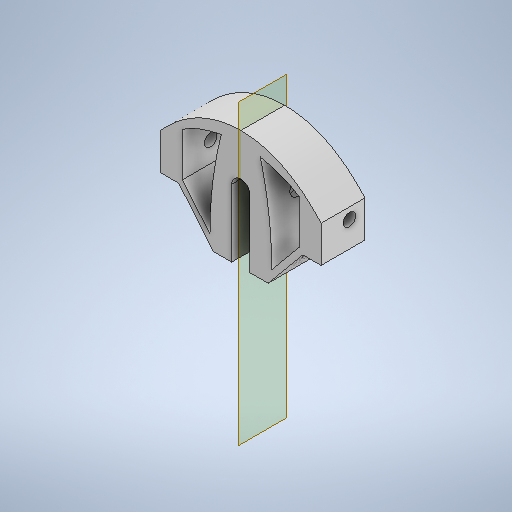
# Autodesk Inventor part: 5th Wheel Body
Saved by Autodesk Inventor 2025 (Build 290162000, 162)
## iProperties
Created: 2024-06-19
Part Number: 5th Wheel Body
Material: 일반
Document SubType Name: Modeling
Designer: unney
Density: 1 g/cm^3
Appearance: 기본값
Author: unney
Autodesk Inventor part; units mm, degrees
ref_plane "YZ Plane" through (0, 0, 0) normal (1, 0, 0) x (0, 1, 0)
ref_plane "XZ Plane" through (0, 0, 0) normal (0, 1, 0) x (-1, 0, 0)
ref_plane "XY Plane" through (0, 0, 0) normal (0, 0, 1) x (1, 0, 0)
sketch "스케치1" plane through (0, 0, 0) normal (0, 0, 1) x (1, 0, 0)
  arc A0 (0, 12.5) -> (-12.5, 0) centre (0, 0) ccw
  line L0 (0, 220.6094) -> (0, -371.145)
  line L1 (-77.086, -220) -> (-110, -35)
  line L2 (-110, -35) -> (-110, 15)
  spline S0 degree 2 poles (-110, 15) (-61.239, 69.4656) (0, 70) knots 0 0 0 1 1 1
  line L3 (-29.7943, 69.74) -> (29.7943, 70.26) construction
  line L4 (-12.5, 0) -> (-12.5, -190)
  line L5 (-12.5, -190) -> (-29.9689, -220)
  line L6 (-29.9689, -220) -> (-77.086, -220)
  arc A1 (12.5, 0) -> (0, 12.5) centre (0, 0) ccw
  line L7 (77.086, -220) -> (110, -35)
  line L8 (110, -35) -> (110, 15)
  spline S1 degree 2 poles (110, 15) (61.239, 69.4656) (0, 70) knots 0 0 0 1 1 1
  line L9 (29.7943, 69.74) -> (-29.7943, 70.26) construction
  line L10 (12.5, 0) -> (12.5, -190)
  line L11 (12.5, -190) -> (29.9689, -220)
  line L12 (29.9689, -220) -> (77.086, -220)
  point P0 (1.2114, -68.8044)
  point P1 (23.5091, 68.2027)
  point P2 (-23.4485, 67.5354)
  point P3 (-1.2114, -68.8044)
  point P4 (-23.5091, 68.2027)
  point P5 (23.4485, 67.5354)
  point P6 (0, 70)
  dimension "d0" = 25
  dimension "d3" = 110
  dimension "d4" = 50
  dimension "d5" = 190
  dimension "d8" = 70
  dimension "d25" = 290
  constraints: 26 end point, 11 symmetric about line, 4 midpoint, 4 point on circle, 2 centre point, 2 point on line, 2 vertical, 1 coincident, 1 horizontal, 1 parallel, 1 perpendicular, 15 other
  measures "d0" diameter of A0
  measures "d3" distance between parallel lines of L0 L2
  measures "d4" distance of L2.end L1.end
  measures "d5" distance of L4.end L4.start
  measures "d8" distance of point (0, 0) point (0, 70)
  measures "d25" distance from line of L12 point (0, 70)
extrude "Wheel Body Initial Extrusion" add sketch "스케치1" along normal mid plane 60
sketch "스케치4" plane through (-12.5, -190, 30) normal (1, 0, 0) x (0, 0, -1)
  line L0 (60, 190) -> (0, 190) projected
  line L1 (60, 190) -> (60, 0) projected
  line L2 (60, 0) -> (0, 0) projected
  line L3 (0, 0) -> (0, 190) projected
  line L4 (0, 190) -> (0, -93.6851)
  line L5 (23, 50) -> (10, 50)
  line L6 (10, 50) -> (10, -48.4584)
  line L7 (10, -10.6044) -> (23, -10.6044)
  line L8 (23, -10.6044) -> (23, -50.5115)
  line L9 (23, -50.5115) -> (0, -50.5115)
  line L10 (53, -93.6851) -> (53, 276.7845)
  line L11 (53, 190) -> (0, 190)
  line L12 (53, 259.8429) -> (0, 259.8429)
  line L13 (0, 259.8429) -> (0, 0)
  point P0 (30, 190)
  dimension "d18" = 13
  dimension "d19" = 140
  dimension "d20" = 7
  constraints: 20 end point, 6 point on line, 4 horizontal, 2 parallel, 2 perpendicular, 1 collinear
  measures "d18" distance of L7.start L7.end
  measures "d19" distance between parallel lines of L5 L0
  measures "d20" distance between parallel lines of L10 L1
sketch "스케치7" plane through (0, 0, 30) normal (0, 0, 1) x (1, 0, 0)
  line L0 (-103, -34.3822) -> (-71.2215, -213)
  line L1 (-71.2215, -213) -> (-34.8207, -213)
  line L2 (-29.9689, -220) -> (-77.086, -220) projected
  line L3 (-34.8207, -213) -> (-19.5, -189.0198)
  line L4 (-19.5, -189.0198) -> (-19.5, 0)
  line L5 (-103, -34.3822) -> (-103, 27.8234)
  line L6 (-103, 27.8234) -> (-55.0885, 51.7889) construction
  line L7 (-55.0885, 51.7889) -> (35.24, 53.8015) construction
  spline S0 degree 2 poles (-103, 27.8234) (-55.0885, 51.7889) (35.24, 53.8015) knots 1 1 1 2 2 2
  line L8 (12.5, -190) -> (12.5, 0) projected
  arc A0 (12.5, 0) -> (-12.5, 0) centre (0, 0) ccw projected
  line L9 (-110, 15) -> (-110, -35) projected
  line L10 (-110, -35) -> (-77.086, -220) projected
  line L11 (-12.5, -190) -> (-12.5, 0) projected
  arc A1 (0, 19.5) -> (-19.5, 0) centre (0, 0) ccw
  line L12 (138.0234, -13.4315) -> (72.0365, -213)
  line L13 (72.0365, -213) -> (34.8207, -213)
  line L14 (34.8207, -213) -> (19.5, -189.0198)
  line L15 (19.5, -189.0198) -> (19.5, 0)
  line L16 (138.0234, -13.4315) -> (173.48, 27.8234)
  line L17 (173.48, 27.8234) -> (125.5685, 51.7889) construction
  line L18 (125.5685, 51.7889) -> (35.24, 53.8015) construction
  spline S1 degree 2 poles (173.48, 27.8234) (125.5685, 51.7889) (35.24, 53.8015) knots 1 1 1 2 2 2
  arc A2 (19.5, 0) -> (0, 19.5) centre (0, 0) ccw
  line L19 (72.0365, 0) -> (72.0365, -130)
  line L20 (106.0933, -110) -> (19.5, -110)
  line L21 (92.8673, -150) -> (19.5, -150)
  point P0 (-103, -3.2794)
  dimension "d40" = 7
  dimension "d42" = 7
  dimension "d43" = 7
  dimension "d44" = 7
  dimension "d53" = 130
  dimension "d54" = 20
  dimension "d57" = 40
  constraints: 26 end point, 4 point on circle, 4 point on line, 3 perpendicular, 2 centre point, 2 vertical, 1 coincident, 1 midpoint, 1 parallel, 9 other
  measures "d40" distance from line of L9 point (-103, -3.279)
  measures "d42" distance between parallel lines of L10 L0
  measures "d43" distance between parallel lines of L2 L1
  measures "d44" distance between parallel lines of L11 L4
  measures "d53" distance of L19.start L19.end
  measures "d54" distance from line of L19.end L20
  measures "d57" distance between parallel lines of L21 L20
extrude "Extrusion Cut for Thickness" [suppressed]
sketch "스케치8" plane through (110, -35, 30) normal (1, 0, 0) x (0, 0, -1)
  line L0 (60, 50) -> (60, 0) projected
  line L1 (60, 50) -> (30, 50)
  line L2 (60, 20) -> (60, 50)
  circle A0 centre (30, 35) radius 8.5
  dimension "d84" = 17
  constraints: 4 end point, 1 centre point, 1 coincident, 1 horizontal
  measures "d84" diameter of A0
extrude "돌출3" [suppressed]
extrude "돌출4" [suppressed]
mirror "미러1" [suppressed]
extrude "돌출5" add sketch "스케치7" against normal blind 23 contours L12 L21 L15 L20
mirror "미러2" about plane through (0, 0, 0) normal (1, 0, 0) of "돌출5"
sketch "스케치21" plane through (0, 0, -30) normal (0, 0, -1) x (-1, 0, 0)
  line L0 (-77.086, -220) -> (-110, -35) projected
  line L1 (-110, -35) -> (-85, -35)
  line L2 (-85, -35) -> (-37.5, -92.3904)
  line L3 (-37.5, -92.3904) -> (-12.5, -92.3904)
  line L4 (-12.5, 0) -> (-12.5, -190) projected
  line L5 (0, 75.7954) -> (0, -227.3908)
  line L6 (110, -35) -> (85, -35)
  line L7 (85, -35) -> (37.5, -92.3904)
  line L8 (37.5, -92.3904) -> (12.5, -92.3904)
  line L9 (-110, -35) -> (-77.086, -220)
  line L10 (-29.9689, -220) -> (-77.086, -220) projected
  line L11 (-12.5, -190) -> (-29.9689, -220) projected
  line L12 (-29.9689, -220) -> (-12.5, -190)
  line L13 (-12.5, -190) -> (-12.5, -92.3904)
  line L14 (12.5, -92.3904) -> (12.5, -190)
  line L15 (29.9689, -220) -> (12.5, -190) projected
  line L16 (12.5, -190) -> (29.9689, -220)
  line L17 (110, -35) -> (77.086, -220) projected
  line L18 (29.9689, -220) -> (77.086, -220)
  line L19 (77.086, -220) -> (110, -35)
  point P0 (0, 0)
  dimension "d80" = 25
  dimension "d81" = 25
  constraints: 28 end point, 4 collinear, 4 symmetric about line, 2 parallel, 1 horizontal, 1 perpendicular, 1 point on line, 1 vertical
  measures "d80" distance of L0.end L1.end
  measures "d81" distance of L2.end L3.end
extrude "돌출9" cut sketch "스케치21" against normal blind 60
sketch "스케치22" plane through (110, 15, 30) normal (1, 0, 0) x (0, 0, -1)
  line L0 (60, -15) -> (0, -15) projected
  circle A0 centre (38.7205, -15) radius 8.5
  point P0 (30, -15)
  dimension "d86" = 17
  constraints: 1 centre point, 1 point on line
  measures "d86" diameter of A0
extrude "돌출10" cut sketch "스케치22" against normal blind 80
sketch "스케치23" plane through (85, -35, -30) normal (0, -1, 0) x (1, 0, 0)
  circle A0 centre (12.5, 45) radius 8.5
  line L0 (25, 0) -> (25, 60) projected
  line L1 (0, 60) -> (25, 60) projected
  point P0 (-85, 30)
  dimension "d89" = 12.5
  dimension "d90" = 17
  dimension "d91" = 15
  constraints: 1 centre point
  measures "d89" distance from line of L0 A0.centre
  measures "d90" diameter of A0
  measures "d91" distance from line of L1 A0.centre
extrude "돌출11" cut sketch "스케치23" against normal blind 40
sketch "스케치24" plane through (12.5, -92.3904, -30) normal (0, -1, 0) x (1, 0, 0)
  circle A0 centre (-37.5, 28) radius 8.5
  circle A1 centre (85, 45) radius 8.5 projected
  line L0 (-50, 0) -> (-50, 60) projected
  point P0 (-12.5, 30)
  dimension "d94" = 17
  dimension "d95" = 17
  dimension "d98" = 12.5
  constraints: 1 centre point
  measures "d94" diameter of A0
  measures "d95" vertical distance of A1.centre A0.centre
  measures "d98" distance from line of L0 A0.centre
extrude "돌출12" cut sketch "스케치24" against normal blind 60 contours A0
ref_plane "작업 평면6" through (0, 0, -30) normal (-1, 0, 0) x (0, 0, 1)
mirror "미러4" about plane through (0, 0, -30) normal (-1, 0, 0) of "돌출10", "돌출11", "돌출12"
sketch "스케치25" plane through (-106.0933, -110, 7) normal (-0.9494, -0.3139, 0) x (0, 0, 1)
  point P0 (-7, 71.1329)
sketch "스케치26" plane through (0, 0, -30) normal (-1, 0, 0) x (0, 0, 1)
  line L0 (94.4532, -100.7618) -> (-29.2969, -100.7618)
  line L1 (-29.2969, -100.7618) -> (-29.2969, -183.2619)
  line L2 (-29.2969, -183.2619) -> (94.4532, -183.2619)
  line L3 (94.4532, -183.2619) -> (94.4532, -100.7618)
  point P0 (30, 0)
  constraints: 8 end point, 2 parallel, 1 horizontal, 1 perpendicular
extrude "돌출13" cut sketch "스케치26" along normal mid plane 574.75
sketch "스케치27" plane through (0, 0, 30) normal (0, 0, 1) x (1, 0, 0)
  line L0 (80, -28.4941) -> (80, 31.156)
  line L1 (89, -35) -> (89, 5) projected
  line L2 (37.5, -92.3904) -> (85, -35) projected
  line L3 (85, -35) -> (85, 52.6509)
  line L4 (33.5, -32.3904) -> (33.5, -92.3904) projected
  line L5 (85, -22.453) -> (42.2581, -74.0946)
  line L6 (110, -8.5) -> (30, -8.5) projected
  line L7 (80, 31.156) -> (61.3028, 45.0673) construction
  line L8 (61.3028, 45.0673) -> (26.6107, 51.872) construction
  spline S0 degree 2 poles (80, 31.156) (61.3028, 45.0673) (26.6107, 51.872) knots 1 1 1 2 2 2
  line L9 (42.2581, -74.0946) -> (42.2581, -8.5) construction
  line L10 (42.2581, -8.5) -> (26.6107, 51.872) construction
  spline S1 degree 2 poles (42.2581, -74.0946) (42.2581, -8.5) (26.6107, 51.872) knots 1 1 1 2 2 2
  point P0 (0, 0)
  dimension "d102" = 8
  dimension "d103" = 5
  constraints: 6 end point, 3 point on line, 2 parallel, 1 perpendicular, 1 vertical, 6 other
  measures "d102" distance between parallel lines of L2 L5
  measures "d103" distance between parallel lines of L3 L0
extrude "돌출14" cut sketch "스케치27" against normal blind 53 contours L5 S1 L6 L0 | L6 S1 S0 L0
mirror "미러5" about plane through (0, 0, -30) normal (-1, 0, 0) of "돌출14"
